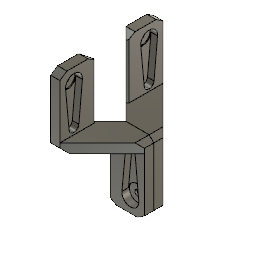
leg1 (Autodesk Fusion 360 design; units mm, degrees)
Autodesk Fusion 360 part; units mm, degrees
sketch "Sketch1" plane through (0, 0, 0) normal (0, 0, 1) x (1, 0, 0)
  line L0 (0, 6) -> (-4, 6)
  line L1 (-4, 6) -> (-4, 18)
  line L2 (-4, 18) -> (0, 18)
  line L3 (0, 18) -> (0, 2)
  line L4 (2, 0) -> (18, 0)
  line L5 (18, 0) -> (18, -4)
  line L6 (18, -4) -> (6, -4)
  line L7 (6, -4) -> (6, 0)
  line L8 (-4, 6) -> (6, -4)
  line L9 (0, 18) -> (18, 0)
  line L10 (3.4142, 0) -> (2.7071, -0.7071)
  line L11 (0, 3.4142) -> (-0.7071, 2.7071)
  constraint horizontal L0
  constraint vertical L1
  constraint horizontal L2
  constraint vertical L3
  constraint horizontal L4
  constraint vertical L5
  constraint horizontal L6
  constraint vertical L7
  constraint coincident L8 L3.end
  constraint coincident L0.start L3
  constraint coincident L8 L4.start
  constraint coincident L7.end L4
  constraint coincident L4 L10.start
  constraint coincident L8 L10.end
  constraint perpendicular L8 L10
  constraint coincident L3 L11.start
  constraint coincident L8 L11.end
  constraint perpendicular L8 L11
extrude "Extrude1" add sketch "Sketch1" along normal mid plane 4 makes body 1
extrude "Extrude2" add sketch "Sketch1" along normal blind 27 contours L0 L3 L8 L11 | L0 L1 L2 L3 bodies 1
extrude "Extrude3" add sketch "Sketch1" against normal blind 27 contours L4 L5 L6 L7 | L4 L7 L8 L10 bodies 1
sketch "Sketch2" plane through (0, 0, 0) normal (1, 0, 0) x (0, 1, 0)
  line L0 (3.4142, 2) -> (18, 2)
  line L1 (18, 2) -> (18, 27)
  line L2 (18, 27) -> (3.4142, 27)
  line L3 (3.4142, 27) -> (3.4142, 2)
  line L4 (18, 27) -> (6, 27)
  line L5 (6, 27) -> (6, 2)
  line L6 (6, 2) -> (18, 2)
  line L7 (18, 2) -> (18, 27)
  circle A0 centre (12, 21) radius 3.6
  circle A1 centre (12, 5) radius 2.1
  line L8 (15.5841, 20.6625) -> (14.0908, 4.8031)
  line L9 (8.4159, 20.6625) -> (9.9092, 4.8031)
  circle A2 centre (12, 21) radius 1.25
  line L10 (6, 27) -> (2.6, 27)
  line L11 (2.6, 27) -> (2.6, 25)
  line L12 (2.6, 25) -> (6, 25)
  line L13 (6, 25) -> (6, 27)
  line L14 (18, 27) -> (15, 27)
  line L15 (15, 27) -> (15, 25)
  line L16 (15, 25) -> (18, 25)
  line L17 (18, 25) -> (18, 27)
  line L18 (18, 25) -> (15, 27)
  line L19 (6, 27) -> (2.6, 25)
  constraint horizontal L4
  constraint vertical L5
  constraint horizontal L6
  constraint vertical L7
  constraint coincident L1.end L2.start
  constraint coincident A0 L8.start
  constraint tangent A0 L8
  constraint coincident A1 L8.end
  constraint tangent A1 L8
  constraint coincident A0 L9.start
  constraint tangent A0 L9
  constraint coincident A1 L9.end
  constraint tangent A1 L9
  constraint horizontal L10
  constraint vertical L11
  constraint horizontal L12
  constraint vertical L13
  constraint horizontal L14
  constraint vertical L15
  constraint horizontal L16
  constraint vertical L17
extrude "Extrude4" cut sketch "Sketch2" against normal blind 2.8 contours A0 A1 L8 L9 | A1 bodies 1
extrude "Extrude5" cut sketch "Sketch2" against normal blind 3.2 contours A0 bodies 1
extrude "Extrude6" cut sketch "Sketch2" against normal blind 4 contours A2 bodies 1
extrude "Extrude7" cut sketch "Sketch2" against normal blind 4 contours L3 L10 L11 L19 | L2 L3 L10 L19 | L1 L2 L4 L7 L14 L17 L18 bodies 1
chamfer "Chamfer1" distance 2 angle 45 1 edges at (-2, 18, -2) on bodies 1
chamfer "Chamfer2" distance 2 angle 45 1 edges at (18, -2, 2) on bodies 1
sketch "Sketch3" plane through (0, 0, 0) normal (0, 1, 0) x (-1, 0, 0)
  line L0 (-3.4142, -2) -> (-18, -2)
  line L1 (-18, -2) -> (-18, -27)
  line L2 (-18, -27) -> (-3.4142, -27)
  line L3 (-3.4142, -27) -> (-3.4142, -2)
  line L4 (-3.4142, -2) -> (-18, -2)
  line L5 (-18, -27) -> (-15, -27)
  circle A0 centre (-12, -21) radius 3.6
  line L6 (-15, -25) -> (-18, -25)
  line L7 (-2.6, -25) -> (-6, -25)
  circle A1 centre (-12, -5) radius 2.1
  line L8 (-6, -25) -> (-6, -27)
  line L9 (-15, -27) -> (-15, -25)
  line L10 (-6, -2) -> (-18, -2)
  line L11 (-18, -27) -> (-6, -27)
  line L12 (-18, -27) -> (-3.4142, -27)
  line L13 (-18, -2) -> (-18, -27)
  circle A2 centre (-12, -21) radius 1.25
  line L14 (-6, -27) -> (-2.6, -27)
  line L15 (-15.5841, -20.6625) -> (-14.0908, -4.8031)
  line L16 (-3.4142, -27) -> (-3.4142, -2)
  line L17 (-6, -27) -> (-6, -2)
  line L18 (-18, -25) -> (-18, -27)
  line L19 (-2.6, -27) -> (-2.6, -25)
  line L20 (-18, -25) -> (-15, -27)
  line L21 (-8.4159, -20.6625) -> (-9.9092, -4.8031)
  line L22 (-6, -27) -> (-2.6, -25)
  line L23 (-18, -2) -> (-18, -27)
  point P0 (0, 0)
  constraint coincident L1.end L2.start
  constraint coincident L15.start A0
  constraint tangent A0 L15
  constraint coincident L15.end A1
  constraint tangent A1 L15
  constraint coincident L21.start A0
  constraint tangent A0 L21
  constraint coincident L21.end A1
  constraint tangent A1 L21
extrude "Extrude8" cut sketch "Sketch3" against normal blind 2.8 contours A0 A1 L15 L21 | A1 bodies 1
extrude "Extrude9" cut sketch "Sketch3" against normal blind 3.2 contours A0 bodies 1
extrude "Extrude10" cut sketch "Sketch3" against normal blind 4 contours A2 bodies 1
extrude "Extrude11" cut sketch "Sketch3" against normal blind 4 contours L3 L14 L16 L19 L22 | L2 L3 L12 L14 L16 L22 | L1 L2 L5 L11 L12 L13 L18 L20 L23 bodies 1
mirror "Mirror1" about plane through (18, -4, 0) normal (0, -1, 0) of bodies 1 makes body 2
named bodies: "leg1", "leg1_mirror"
